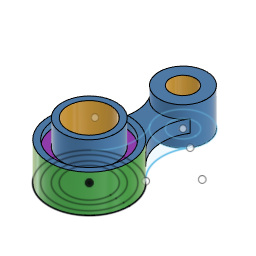
Ex 5 v2 (Autodesk Fusion 360 design; units mm, degrees)
Autodesk Fusion 360 part; units mm, degrees
sketch "Esboço1" plane through (0, 0, 0) normal (0, 0, 1) x (1, 0, 0)
  circle A0 centre (0, 0) radius 17
  circle A1 centre (0, 0) radius 21.5
  circle A2 centre (0, 0) radius 27.5
  circle A3 centre (0, 0) radius 32
  circle A4 centre (0, 75) radius 10
  circle A5 centre (0, 75) radius 19
  arc A6 (-21.4646, 23.7333) -> (-15.9932, 64.7425) centre (-42.9292, 47.4667) ccw
  arc A7 (15.9932, 64.7425) -> (21.4646, 23.7333) centre (42.9292, 47.4667) ccw
  dimension "d1" = 34
  dimension "d2" = 43
  dimension "d3" = 55
  dimension "d4" = 64
  dimension "d5" = 75
  dimension "d6" = 20
  dimension "d7" = 38
  dimension "d8" = 64
  constraint coincident A0.centre A1.centre
  constraint concentric A0 A1
  constraint concentric A0 A2
  constraint concentric A0 A3
  constraint concentric A4 A5
  constraint tangent A5 A6
  constraint tangent A3 A6
  constraint coincident A5 A6.end
  constraint coincident A3 A6.start
  measures "d1" diameter of A0
  measures "d2" diameter of A1
  measures "d3" diameter of A2
  measures "d4" diameter of A3
  measures "d5" distance of A0.centre A4.centre
  measures "d6" diameter of A4
  measures "d7" diameter of A5
  measures "d8" diameter of A6
extrude "Extrusão1" add sketch "Esboço1" along normal blind 30 contours A5 makes body 1
extrude "Extrusão2" add sketch "Esboço1" along normal blind 30 separate body contours A3 makes body 2
extrude "Extrusão3" add sketch "Esboço1" along normal blind 25 contours A2 bodies 2
extrude "Extrusão4" add sketch "Esboço1" along normal blind 45 contours A1 bodies 2
extrude "Extrusão5" add sketch "Esboço1" along normal blind 20 contours A3 A5 A6 A7 bodies 1 2
extrude "Extrusão6" cut sketch "Esboço1" along normal blind 10 contours A3 A5 A6 A7 bodies 1
